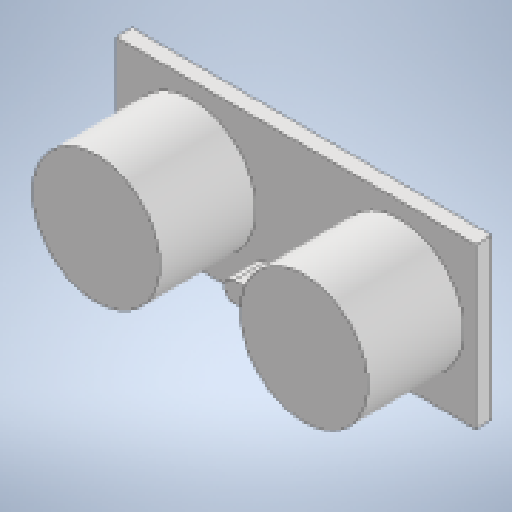
# Autodesk Inventor part: distance
Saved by Autodesk Inventor 2024 (Build 280153000, 153)
## iProperties
Created: 2024-03-14
Part Number: distance
Material: Générique
Document SubType Name: Modeling
Designer: phaly
Density: 1 g/cm^3
Appearance: Par défaut
Author: phaly
Autodesk Inventor part; units mm, degrees
ref_plane "YZ Plane" through (0, 0, 0) normal (1, 0, 0) x (0, 1, 0)
ref_plane "XZ Plane" through (0, 0, 0) normal (0, 1, 0) x (-1, 0, 0)
ref_plane "XY Plane" through (0, 0, 0) normal (0, 0, 1) x (1, 0, 0)
sketch "Esquisse1" plane through (0, 0, 0) normal (0, 0, 1) x (1, 0, 0)
  line L0 (0, 20) -> (45, 20)
  line L1 (45, 20) -> (45, 0)
  line L2 (45, 0) -> (0, 0)
  line L3 (0, 0) -> (0, 20)
  line L4 (-9, 0) -> (54, 0) projected
  line L5 (0, -4) -> (0, 24) projected
  point P0 (0, 0)
  dimension "d0" = 20
  dimension "d1" = 45
  constraints: 8 end point, 2 collinear, 2 parallel, 1 horizontal, 1 perpendicular
  measures "d0" distance of L0.end L1.end
  measures "d1" distance of L0.start L0.end
extrude "Extrusion1" add sketch "Esquisse1" along normal blind 2
sketch "Esquisse2" plane through (0, 0, 2) normal (0, 0, 1) x (1, 0, 0)
  circle A0 centre (9.5, 10) radius 8
  circle A1 centre (35.5, 10) radius 8
  line L0 (0, 10) -> (43.5, 10)
  line L1 (45, 20) -> (0, 20) projected
  line L2 (0, 20) -> (0, 0) projected
  dimension "d6" = 16
  dimension "d4" = 10
  dimension "d5" = 16
  dimension "d7" = 26
  dimension "d8" = 9.5
  constraints: 2 end point, 2 point on line, 1 centre point, 1 horizontal, 1 horizontal alignment, 1 midpoint, 2 other
  measures "d4" distance between parallel lines of L1 L0
  measures "d5" diameter of A0
  measures "d7" distance of point (35.5, 10) A0.centre
  measures "d8" distance from line of L2 A0.centre
extrude "Extrusion2" add sketch "Esquisse2" along normal blind 12
sketch "Esquisse3" plane through (0, 0, 2) normal (0, 0, 1) x (1, 0, 0)
  line L0 (18.75, 3.75) -> (26.25, 3.75) construction
  line L1 (18.75, 2.5) -> (26.25, 2.5)
  line L2 (26.25, 5) -> (18.75, 5)
  arc A0 (18.75, 5) -> (18.75, 2.5) centre (18.75, 3.75) ccw
  arc A1 (26.25, 2.5) -> (26.25, 5) centre (26.25, 3.75) ccw
  line L3 (45, 0) -> (45, 20) projected
  line L4 (0, 0) -> (45, 0) projected
  point P0 (22.5, 3.75)
  point P1 (27.5, 3.75)
  point P2 (17.5, 3.75)
  dimension "d11" = 10
  dimension "d12" = 2.5
  dimension "d13" = 22.5
  dimension "d14" = 5
  constraints: 8 end point, 6 point on circle, 4 tangent, 2 centre point, 1 horizontal, 1 midpoint, 1 parallel
  measures "d11" distance of point (27.5, 3.75) point (17.5, 3.75)
  measures "d12" distance between parallel lines of L1 L2
  measures "d13" distance from line of L3 point (22.5, 3.75)
  measures "d14" distance between parallel lines of L4 L2
extrude "Extrusion3" add sketch "Esquisse3" along normal blind 4
equation "\"d6\" = d5"
